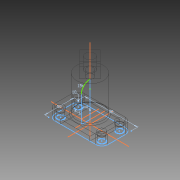
# Autodesk Inventor part: Piesa 2 3D
Saved by Autodesk Inventor 2011 SP2 (Build 150309200, 309)
## iProperties
Created: 2023-03-06
Part Number: Piesa 2 3D
Document SubType Name: Modeling
Designer: utilizator
Density: 1 g/cm^3
Author: utilizator
Autodesk Inventor part; units mm, degrees
ref_plane "YZ Plane" through (0, 0, 0) normal (1, 0, 0) x (0, 1, 0)
ref_plane "XZ Plane" through (0, 0, 0) normal (0, 1, 0) x (-1, 0, 0)
ref_plane "XY Plane" through (0, 0, 0) normal (0, 0, 1) x (1, 0, 0)
sketch "Sketch1" plane through (0, 0, 0) normal (0, 0, 1) x (1, 0, 0)
  line L0 (-65.8995, 0) -> (65.8995, 0) projected
  line L1 (0, -37.8995) -> (0, 37.8995) projected
  line L2 (-45, 0) -> (-45, 15)
  line L3 (-35, 25) -> (0, 25)
  arc A0 (-35, 25) -> (-45, 15) centre (-35, 15) ccw
  circle A1 centre (-35, 15) radius 5
  circle A2 centre (-35, 15) radius 6
  circle A3 centre (-35, -15) radius 6
  circle A4 centre (35, 15) radius 6
  circle A5 centre (35, -15) radius 6
  circle A6 centre (-35, -15) radius 5
  circle A7 centre (35, 15) radius 5
  circle A8 centre (35, -15) radius 5
  line L4 (-45, 0) -> (-45, -15)
  line L5 (-35, -25) -> (0, -25)
  arc A9 (-45, -15) -> (-35, -25) centre (-35, -15) ccw
  line L6 (45, 0) -> (45, 15)
  line L7 (35, 25) -> (0, 25)
  arc A10 (45, 15) -> (35, 25) centre (35, 15) ccw
  line L8 (35, -25) -> (0, -25)
  arc A11 (35, -25) -> (45, -15) centre (35, -15) ccw
  line L9 (45, 0) -> (45, -15)
  point P0 (0, 0)
  point P1 (-45, 25)
  point P2 (-45, -25)
  point P3 (45, 25)
  dimension "d3" = 50
  dimension "d4" = 90
  dimension "d6" = 10
  dimension "d10" = 5
  dimension "d14" = 6
  constraints: 19 symmetric about line, 16 end point, 12 centre point, 8 point on circle, 3 point on line, 2 coincident, 2 tangent, 1 parallel, 1 perpendicular, 1 vertical alignment, 9 other
  measures "d3" distance of point (-45, -25) point (-45, 25)
  measures "d4" distance of point (45, 25) point (-45, 25)
  measures "d6" radius of A0
  measures "d10" radius of A1
  measures "d14" radius of A2
extrude "Extrusion1" add sketch "Sketch1" along normal blind 15 contours L2 A0 L3 L1 L0 | L0 L1 L5 A9 L4 | L1 L7 A10 L6 L0 | L0 L9 A11 L8 L1
extrude "Extrusion2" add sketch "Sketch1" along normal blind 10 contours A2 | A3 | A4 | A5
sketch "Sketch2" plane through (-35, -25, 0) normal (0, -1, 0) x (1, 0, 0)
  line L0 (0, 0) -> (70, 0) projected
  line L1 (35, -3) -> (35, 18) projected
  line L2 (10, 7) -> (10, 0)
  line L3 (60, 7) -> (60, 0)
  line L4 (10, 7) -> (60, 7)
  line L5 (10, 0) -> (60, 0)
  point P0 (35, 0)
  dimension "d20" = 7
  dimension "d21" = 50
  constraints: 8 end point, 2 perpendicular, 2 symmetric about line, 1 collinear, 1 point on line
  measures "d20" distance of L2.start L2.end
  measures "d21" distance of L3.start L2.start
extrude "Extrusion3" cut sketch "Sketch2" against normal blind 50
sketch "Sketch3" plane through (0, 0, 15) normal (0, 0, 1) x (1, 0, 0)
  circle A0 centre (0, 0) radius 22.5
  dimension "d24" = 22.5
  constraints: 1 centre point, 1 coincident
  measures "d24" radius of A0
extrude "Extrusion4" add sketch "Sketch3" along normal blind 60
sketch "Sketch4" plane through (0, 0, 75) normal (0, 0, 1) x (1, 0, 0)
  circle A0 centre (0, 0) radius 22.5 projected
  line L0 (-17.6777, 0) -> (0, 17.6777)
  line L1 (0, 17.6777) -> (17.6777, 0)
  line L2 (17.6777, 0) -> (0, -17.6777)
  line L3 (0, -17.6777) -> (-17.6777, 0)
  dimension "d30" = 25
  dimension "d31" = 25
  dimension "d32" = 25
  dimension "d33" = 25
  constraints: 8 end point, 2 vertical alignment, 1 horizontal alignment, 1 perpendicular
  measures "d30" distance of L0.start L0.end
  measures "d31" distance of L0.end L1.end
  measures "d32" distance of L1.end L2.end
  measures "d33" distance of L2.end L0.start
extrude "Extrusion5" add sketch "Sketch4" along normal blind 25 contours L0 L1 L2 L3
fillet "Fillet1" radius 2 1 edges at (-22.5, 0, 15)
hole "Hole1" at (0, 0, 100) direction (0, 0, -1) diameter 16 depth 20
hole "Hole2" at (0, 0, 80) direction (0, 0, -1) diameter 12 depth 10 tip angle 118
sketch "Sketch5" plane through (0, 0, 0) normal (1, 0, 0) x (0, 1, 0)
  line L0 (0, -20) -> (0, 120) projected
  line L1 (-25, 7) -> (25, 7) projected
  line L2 (-35, 0) -> (35, 0) projected
  line L3 (-15, 8.1453) -> (-15, 51.4254)
  line L4 (-15, 15) -> (15, 15) projected
  arc A0 (0, 66.4254) -> (-15, 51.4254) centre (0, 51.4254) ccw
  line L5 (0, 66.4254) -> (0, 7)
  line L6 (0, 7) -> (-15, 7)
  line L7 (0, 66.4254) -> (0, 7)
  point P0 (0, 0)
  point P1 (0, 15)
  point P2 (0, 15)
  point P3 (0, 15)
  dimension "d57" = 15
  constraints: 8 end point, 4 midpoint, 2 perpendicular, 2 point on circle, 2 point on line, 2 vertical alignment, 1 centre point, 1 collinear, 1 tangent
  measures "d57" radius of A0
body "Solid1"
